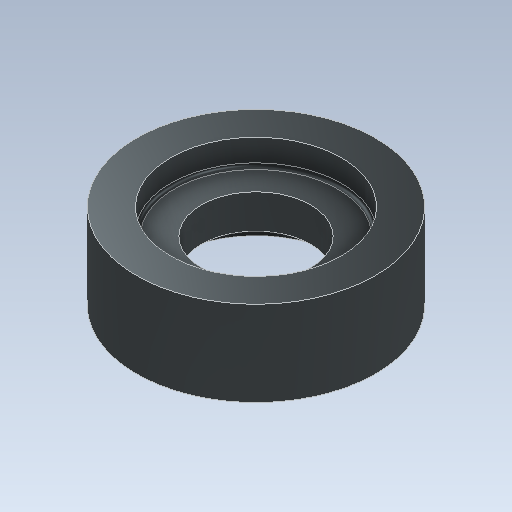
# Autodesk Inventor part: Корпус сальника перегородка 1_CPY
Saved by Autodesk Inventor 2021 (Build 250183000, 183)
## iProperties
Created: 2020-11-17
Part Number: Корпус сальника перегородка 1_CPY
Material: Чугун, серый
Document SubType Name: Modeling
Designer: Тимоха
Mass: 3362.4 g
Surface Area: 592.479 cm^2
Volume: 470.265 cm^3
Density: 7.15 g/cm^3
Appearance: Чугун серый
Author: Тимоха
Autodesk Inventor part; units mm, degrees
ref_plane "YZ Plane" through (0, 0, 0) normal (1, 0, 0) x (0, 1, 0)
ref_plane "XZ Plane" through (0, 0, 0) normal (0, 1, 0) x (-1, 0, 0)
ref_plane "XY Plane" through (0, 0, 0) normal (0, 0, 1) x (1, 0, 0)
sketch "Эскиз1" plane through (0, 0, 0) normal (0, 0, 1) x (1, 0, 0)
  line L0 (0, 0) -> (0, 10)
  line L1 (0, 10) -> (50, 10)
  line L2 (50, 10) -> (50, 25)
  line L3 (50, 25) -> (70, 25)
  line L4 (70, 25) -> (70, 3)
  line L5 (0, 0) -> (4.3397, 0)
  line L6 (0, -10) -> (50, -10)
  line L7 (50, -10) -> (50, -25)
  line L8 (50, -25) -> (70, -25)
  line L9 (70, -25) -> (70, 3)
  line L10 (0, 10) -> (32, 10)
  line L11 (32, 10) -> (32, -10)
  dimension "d0" = 10
  dimension "d1" = 50
  dimension "d2" = 15
  dimension "d3" = 20
  dimension "d4" = 32
  constraints: 24 end point, 4 symmetric about line, 3 perpendicular, 2 horizontal, 2 point on line, 2 vertical
  measures "d0" distance of L0.start L0.end
  measures "d1" distance of L0.end L1.end
  measures "d2" distance of L1.end L2.end
  measures "d3" distance of L2.end L3.end
  measures "d4" distance of L0.end L10.end
revolve "Вращение1" add sketch "Эскиз1" angle 360 about axis through (0, 0, 0) along (0, 1, 0)
fillet "Сопряжение1" radius 2 2 edges at (-50, 10, 0) (-50, -10, 0)
